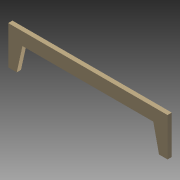
# Autodesk Inventor part: ridgidizer
Saved by Autodesk Inventor 2012 (Build 160160000, 160)
## iProperties
Created: 2013-05-09
Part Number: ridgidizer
Material: Default
Document SubType Name: Modeling
Designer: Fabian
Density: 1 g/cm^3
Author: Fabian
Autodesk Inventor part; units mm, degrees
ref_plane "YZ Plane" through (0, 0, 0) normal (1, 0, 0) x (0, 1, 0)
ref_plane "XZ Plane" through (0, 0, 0) normal (0, 1, 0) x (-1, 0, 0)
ref_plane "XY Plane" through (0, 0, 0) normal (0, 0, 1) x (1, 0, 0)
sketch "Sketch1" plane through (0, 0, 0) normal (0, 0, 1) x (1, 0, 0)
  line L0 (-20.8392, 159.2122) -> (690.3608, 159.2122)
  line L1 (690.3608, 159.2122) -> (690.3608, -12.2378)
  line L2 (690.3608, -12.2378) -> (-20.8392, -12.2378)
  line L3 (-20.8392, -12.2378) -> (-20.8392, 159.2122)
  point P0 (0, 0)
  dimension "d0" = 171.45
  dimension "d1" = 711.2
  constraints: 8 end point, 2 parallel, 1 horizontal, 1 perpendicular
  measures "d0" distance of L2.end L0.start
  measures "d1" distance of L1.end L2.end
extrude "Extrusion1" add sketch "Sketch1" along normal blind 19.05
sketch "Sketch2" plane through (0, 0, 19.05) normal (0, 0, 1) x (1, 0, 0)
  line L0 (690.3608, 159.2122) -> (690.3608, -12.2378) projected
  line L1 (-20.8392, -12.2378) -> (-20.8392, 159.2122) projected
  line L2 (690.3608, -12.2378) -> (-20.8392, -12.2378) projected
  line L3 (42.6608, 102.0622) -> (626.8608, 102.0622)
  line L4 (626.8608, 102.0622) -> (626.8608, -12.2378)
  line L5 (626.8608, -12.2378) -> (42.6608, -12.2378)
  line L6 (42.6608, -12.2378) -> (42.6608, 102.0622)
  line L7 (42.6608, 102.0622) -> (17.2608, -12.2378)
  line L8 (626.8608, 102.0622) -> (652.2608, -12.2378)
  point P0 (0, 0)
  dimension "d4" = 25.4
  dimension "d5" = 25.4
  dimension "d6" = 38.1
  dimension "d7" = 38.1
  dimension "d10" = 114.3
  constraints: 12 end point, 3 point on line, 2 parallel, 1 horizontal, 1 perpendicular
  measures "d4" distance of L5.end L7.end
  measures "d5" distance of L8.end L4.end
  measures "d6" distance from line of L1 L7.end
  measures "d7" distance from line of L0 L8.end
  measures "d10" distance between parallel lines of L2 L3
extrude "Extrusion2" cut sketch "Sketch2" against normal blind 19.05
body "Solid1"
